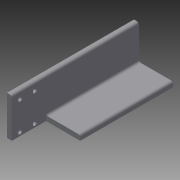
# Autodesk Inventor part: lbeam final
Saved by Autodesk Inventor 2015 (Build 190159000, 159)
## iProperties
Created: 2015-02-21
Part Number: lbeam final
Material: Generic
Document SubType Name: Modeling
Designer: chapale16
Density: 1 g/cm^3
Appearance: Default
Author: chapale16
Autodesk Inventor part; units mm, degrees
ref_plane "YZ Plane" through (0, 0, 0) normal (1, 0, 0) x (0, 1, 0)
ref_plane "XZ Plane" through (0, 0, 0) normal (0, 1, 0) x (-1, 0, 0)
ref_plane "XY Plane" through (0, 0, 0) normal (0, 0, 1) x (1, 0, 0)
sketch "Sketch1" plane through (0, 0, 0) normal (0, 0, 1) x (1, 0, 0)
  line L0 (0, 0) -> (6.35, 0)
  line L1 (6.35, 0) -> (6.35, 50.8)
  line L2 (6.35, 50.8) -> (0, 50.8)
  line L3 (0, 50.8) -> (0, 0)
  line L4 (0, 0) -> (50.8, 0)
  line L5 (50.8, 0) -> (50.8, 6.35)
  line L6 (50.8, 6.35) -> (0, 6.35)
  line L7 (0, 6.35) -> (0, 0)
  dimension "d0" = 6.35
  dimension "d1" = 50.8
  dimension "d2" = 50.8
  dimension "d3" = 6.35
  constraints: 16 end point, 4 parallel, 2 horizontal, 2 perpendicular
  measures "d0" distance of L2.end L1.end
  measures "d1" distance of L1.end L0.end
  measures "d2" distance of L6.end L5.end
  measures "d3" distance of L5.end L4.end
extrude "Extrusion1" add sketch "Sketch1" along normal blind 165.1
fillet "Fillet1" radius 3.175 3 edges at (6.35, 50.8, 82.55) (6.35, 6.35, 82.55) (50.8, 6.35, 82.55)
sketch "Sketch2" plane through (0, 0, 0) normal (0, -1, 0) x (1, 0, 0)
  line L0 (0, 165.1) -> (50.8, 165.1) projected
  line L1 (0, 0) -> (0, 165.1) projected
  line L2 (0, 0) -> (50.8, 0) projected
  line L3 (50.8, 0) -> (50.8, 165.1) projected
  line L4 (50.8, 165.1) -> (50.8, 0) projected
  line L5 (6.35, 165.1) -> (50.8, 165.1)
  line L6 (50.8, 165.1) -> (50.8, 120.65)
  line L7 (50.8, 120.65) -> (6.35, 120.65)
  line L8 (6.35, 120.65) -> (6.35, 165.1)
  dimension "d7" = 44.45
  constraints: 8 end point, 2 parallel, 1 horizontal, 1 perpendicular, 1 point on line
  measures "d7" distance of L5.end L6.end
extrude "Extrusion2" cut sketch "Sketch2" against normal blind 165.1 contours L0 L3 L7 L8
sketch "Sketch3" plane through (0, 0, 0) normal (-1, 0, 0) x (0, 0, 1)
  circle A0 centre (135.255, 4.445) radius 2.54 projected
  circle A1 centre (154.305, 4.445) radius 2.54 projected
  circle A2 centre (154.305, 41.275) radius 2.54 projected
  circle A3 centre (135.255, 41.275) radius 2.54 projected
  line L0 (124.46, 45.72) -> (124.46, 0) projected
  line L1 (144.78, 45.72) -> (124.46, 45.72) projected
  line L2 (165.1, 45.72) -> (144.78, 45.72) projected
  line L3 (165.1, 0) -> (165.1, 45.72) projected
  line L4 (124.46, 0) -> (165.1, 0) projected
  point P0 (0, 0)
extrude "Extrusion3" cut sketch "Sketch3" against normal blind 165.1 contours A0 | A1 | A2 | A3
body "Solid1"
